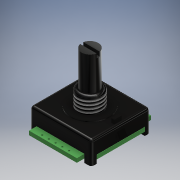
# Autodesk Inventor part: Bourns ACE 128
Saved by Autodesk Inventor 2017 SP1 (Build 210196100, 196)
## iProperties
Created: 2018-01-09
Part Number: Bourns ACE 128
Material: ABS Plastic
Document SubType Name: Modeling
Designer: Zach
Density: 1.06 g/cm^3
Appearance: Glossy - Black
Author: Zach
Autodesk Inventor part; units mm, degrees
ref_plane "YZ Plane" through (0, 0, 0) normal (1, 0, 0) x (0, 1, 0)
ref_plane "XZ Plane" through (0, 0, 0) normal (0, 1, 0) x (-1, 0, 0)
ref_plane "XY Plane" through (0, 0, 0) normal (0, 0, 1) x (1, 0, 0)
sketch "Sketch1" plane through (0, 0, 0) normal (0, 0, 1) x (1, 0, 0)
  line L0 (0, 0) -> (18.04, 0)
  line L1 (18.04, 0) -> (18.04, 27.94) construction
  line L2 (18.04, 27.94) -> (0, 27.94)
  line L3 (0, 27.94) -> (0, 0) construction
  circle A0 centre (9.02, 26.94) radius 0.32
  circle A1 centre (6.48, 26.94) radius 0.32
  circle A2 centre (3.94, 26.94) radius 0.32
  circle A3 centre (11.56, 26.94) radius 0.32
  circle A4 centre (14.1, 26.94) radius 0.32
  circle A5 centre (9.02, 1) radius 0.32
  circle A6 centre (6.48, 1) radius 0.32
  circle A7 centre (3.94, 1) radius 0.32
  circle A8 centre (11.56, 1) radius 0.32
  circle A9 centre (14.1, 1) radius 0.32
  line L4 (-2.665, 23.07) -> (20.705, 23.07) construction
  line L5 (20.705, 23.07) -> (20.705, 4.87) construction
  line L6 (20.705, 4.87) -> (-2.665, 4.87) construction
  line L7 (-2.665, 4.87) -> (-2.665, 23.07) construction
  line L8 (0, 27.94) -> (0, 23.07)
  line L9 (0, 23.07) -> (-2.665, 23.07)
  line L10 (-2.665, 23.07) -> (-2.665, 4.87)
  line L11 (-2.665, 4.87) -> (0, 4.87)
  line L12 (0, 0) -> (0, 4.87)
  line L13 (18.04, 0) -> (18.04, 4.87)
  line L14 (18.04, 4.87) -> (20.705, 4.87)
  line L15 (20.705, 4.87) -> (20.705, 23.07)
  line L16 (20.705, 23.07) -> (18.04, 23.07)
  line L17 (18.04, 23.07) -> (18.04, 27.94)
  point P0 (9.02, 27.94)
  point P1 (9.02, 23.07)
  point P2 (18.04, 13.97)
  point P3 (20.705, 13.97)
  dimension "d0" = 18.04
  dimension "d1" = 27.94
  dimension "d2" = 0.64
  dimension "d3" = 0.64
  dimension "d4" = 2.54
  dimension "d5" = 0.64
  dimension "d6" = 0.64
  dimension "d7" = 0.64
  dimension "d8" = 2.54
  dimension "d9" = 2.54
  dimension "d10" = 2.54
  dimension "d11" = 1
  dimension "d12" = 0.64
  dimension "d13" = 0.64
  dimension "d14" = 2.54
  dimension "d15" = 0.64
  dimension "d16" = 0.64
  dimension "d17" = 0.64
  dimension "d18" = 2.54
  dimension "d19" = 2.54
  dimension "d20" = 2.54
  dimension "d21" = 1
  dimension "d24" = 23.37
  dimension "d25" = 18.2
  constraints: 36 end point, 10 centre point, 9 horizontal alignment, 8 point on line, 4 collinear, 4 midpoint, 4 parallel, 4 perpendicular, 3 vertical alignment, 2 horizontal
  measures "d0" distance of L2.end L1.end
  measures "d1" distance of L1.end L0.end
  measures "d2" diameter of A0
  measures "d3" diameter of A1
  measures "d4" distance of A0.centre A1.centre
  measures "d5" diameter of A2
  measures "d6" diameter of A3
  measures "d7" diameter of A4
  measures "d8" distance of A3.centre A0.centre
  measures "d9" distance of A4.centre A3.centre
  measures "d10" distance of A2.centre A1.centre
  measures "d11" distance from line of L2 A2.centre
  measures "d12" diameter of A5
  measures "d13" diameter of A6
  measures "d14" distance of A5.centre A6.centre
  measures "d15" diameter of A7
  measures "d16" diameter of A8
  measures "d17" diameter of A9
  measures "d18" distance of A8.centre A5.centre
  measures "d19" distance of A9.centre A8.centre
  measures "d20" distance of A7.centre A6.centre
  measures "d21" distance from line of L0 A5.centre
  measures "d24" distance of L5.end L6.end
  measures "d25" distance of L4.end L5.end
extrude "Extrusion1" add sketch "Sketch1" along normal blind 1.5
sketch "Sketch2" plane through (0, 0, 1.5) normal (0, 0, 1) x (1, 0, 0)
  line L0 (-2.565, 25.07) -> (20.605, 25.07)
  line L1 (20.605, 25.07) -> (20.605, 2.87)
  line L2 (20.605, 2.87) -> (-2.565, 2.87)
  line L3 (-2.565, 2.87) -> (-2.565, 25.07)
  line L4 (-2.665, 23.07) -> (-2.665, 4.87) projected
  line L5 (20.705, 4.87) -> (20.705, 23.07) projected
  line L6 (18.04, 27.94) -> (0, 27.94) projected
  point P0 (0, 0)
  point P1 (9.02, 25.07)
  point P2 (9.02, 27.94)
  dimension "d27" = 22.2
  dimension "d30" = 0.1
  constraints: 8 end point, 2 midpoint, 2 parallel, 1 horizontal, 1 perpendicular, 1 vertical alignment
  measures "d27" distance of L0.end L1.end
  measures "d30" distance between parallel lines of L5 L1
extrude "Extrusion2" add sketch "Sketch2" along normal blind 5.51
sketch "Sketch3" plane through (0, 0, 1.5) normal (0, 0, -1) x (-1, 0, 0)
  line L0 (0, 23.07) -> (2.565, 23.07) projected
  line L1 (2.565, 23.07) -> (2.565, 25.07) projected
  line L2 (2.565, 25.07) -> (0, 25.07) projected
  line L3 (0, 25.07) -> (0, 23.07) projected
  line L4 (0, 4.87) -> (0, 2.87) projected
  line L5 (0, 2.87) -> (2.565, 2.87) projected
  line L6 (2.565, 2.87) -> (2.565, 4.87) projected
  line L7 (2.565, 4.87) -> (0, 4.87) projected
  line L8 (-20.605, 23.07) -> (-18.04, 23.07) projected
  line L9 (-18.04, 23.07) -> (-18.04, 25.07) projected
  line L10 (-18.04, 25.07) -> (-20.605, 25.07) projected
  line L11 (-20.605, 25.07) -> (-20.605, 23.07) projected
  line L12 (-18.04, 2.87) -> (-18.04, 4.87) projected
  line L13 (-18.04, 4.87) -> (-20.605, 4.87) projected
  line L14 (-20.605, 4.87) -> (-20.605, 2.87) projected
  line L15 (-20.605, 2.87) -> (-18.04, 2.87) projected
  point P0 (0, 0)
extrude "Extrusion3" add sketch "Sketch3" along normal blind 3
sketch "Sketch4" plane through (0, 0, 7.01) normal (0, 0, 1) x (1, 0, 0)
  circle A0 centre (9.02, 13.97) radius 4.5
  line L0 (20.605, 25.07) -> (-2.565, 25.07) construction
  line L1 (-2.565, 25.07) -> (-2.565, 2.87) construction
  line L2 (-2.565, 2.87) -> (20.605, 2.87) construction
  line L3 (20.605, 2.87) -> (20.605, 25.07) construction
  point P0 (0, 0)
  point P1 (9.02, 25.07)
  point P2 (20.605, 13.97)
  dimension "d33" = 9
  constraints: 2 midpoint, 1 centre point, 1 horizontal alignment, 1 vertical alignment
  measures "d33" diameter of A0
extrude "Extrusion4" add sketch "Sketch4" along normal blind 6.35
sketch "Sketch5" plane through (9.02, 13.97, 13.36) normal (0, 0, 1) x (1, 0, 0)
  circle A0 centre (0, 0) radius 3.16
  circle A1 centre (0, 0) radius 4.5 construction
  point P0 (-9.02, -13.97)
  dimension "d36" = 6.32
  constraints: 1 centre point, 1 coincident
  measures "d36" diameter of A0
extrude "Extrusion5" add sketch "Sketch5" along normal blind 12.7
sketch "Sketch6" plane through (9.02, 13.97, 26.06) normal (0, 0, 1) x (1, 0, 0)
  line L0 (-3.16, 0.595) -> (3.16, 0.595)
  line L1 (3.16, 0.595) -> (3.16, -0.595)
  line L2 (3.16, -0.595) -> (-3.16, -0.595)
  line L3 (-3.16, -0.595) -> (-3.16, 0.595)
  circle A0 centre (0, 0) radius 3.16 construction
  point P0 (-9.02, -13.97)
  point P1 (3.16, 0)
  point P2 (0, 0.595)
  dimension "d39" = 1.19
  constraints: 8 end point, 2 horizontal alignment, 2 midpoint, 2 parallel, 1 horizontal, 1 perpendicular, 1 vertical alignment, 1 other
  measures "d39" distance of L0.end L1.end
extrude "Extrusion6" cut sketch "Sketch6" against normal blind 1.6
thread "Thread1" size "M9x1.25" class "6g" standard "ANSI Metric M Profile" full length
fillet "Fillet1" radius 1 1 edges at (4.52, 13.97, 13.36)
fillet "Fillet2" radius 1 4 edges at (20.605, 2.87, 2.755) (-2.565, 2.87, 2.755) (-2.565, 25.07, 2.755) (20.605, 25.07, 2.755)
fillet "Fillet3" radius 1 8 edges at (-2.2721, 24.7771, 7.01) (-2.565, 13.97, 7.01) (-2.2721, 3.1629, 7.01) (9.02, 2.87, 7.01) (20.3121, 3.1629, 7.01) (20.605, 13.97, 7.01) (20.3121, 24.7771, 7.01) (9.02, 25.07, 7.01)
ref_plane "Work Plane1" through (0, 13.97, 1.5) normal (0, 1, 0) x (1, 0, 0)
sketch "Sketch8" plane through (0, 13.97, 1.5) normal (0, 1, 0) x (1, 0, 0)
  line L0 (19.605, -1.51) -> (21.605, -1.51)
  line L1 (19.605, 3) -> (19.605, -4.51) construction
  line L2 (19.605, -1.51) -> (19.605, -5.51)
  line L3 (0, 1.5) -> (18.04, 1.5) construction
  line L4 (9.02, 1.5) -> (9.02, -5.51) construction
  line L5 (19.605, -5.51) -> (-1.565, -5.51) construction
  line L6 (21.605, -1.51) -> (19.605, -5.51)
  line L7 (-1.565, -1.51) -> (-3.565, -1.51)
  line L8 (-1.565, -1.51) -> (-1.565, -5.51)
  line L9 (-3.565, -1.51) -> (-1.565, -5.51)
  dimension "d47" = 2
  dimension "d48" = 4
  constraints: 14 end point, 3 symmetric about line, 2 vertical, 1 horizontal, 1 midpoint, 1 point on line
  measures "d47" distance of L0.start L0.end
  measures "d48" distance of L2.end L0.start
extrude "Extrusion7" add sketch "Sketch8" along normal mid plane 2.79
sketch "Sketch9" plane through (0, 13.97, 1.5) normal (0, 1, 0) x (1, 0, 0)
  line L0 (-1.565, -5.51) -> (19.605, -5.51) projected
  line L1 (19.605, -5.51) -> (18.415, -5.51)
  line L2 (18.415, -5.51) -> (18.415, -7.03)
  line L3 (18.415, -7.03) -> (19.605, -7.03)
  line L4 (19.605, -7.03) -> (19.605, -5.51)
  point P0 (0, 1.5)
  dimension "d51" = 1.52
  dimension "d52" = 1.19
  constraints: 8 end point, 2 parallel, 1 horizontal, 1 perpendicular
  measures "d51" distance of L2.end L1.end
  measures "d52" distance of L2.end L3.end
extrude "Extrusion8" add sketch "Sketch9" along normal mid plane 2.79
sketch "Sketch10" plane through (0, 0, 7.01) normal (0, 0, 1) x (1, 0, 0)
  circle A0 centre (9.02, 13.97) radius 4.5 projected
  circle A1 centre (9.02, 13.97) radius 7.35
  point P0 (0, 0)
  dimension "d55" = 14.7
  constraints: 1 centre point, 1 coincident
  measures "d55" diameter of A1
extrude "Extrusion9" add sketch "Sketch10" along normal blind 0.25 contours A0 | A1
equation "\"d2\" = d5"
equation "\"d3\" = d5"
equation "\"d6\" = d5"
equation "\"d7\" = d5"
equation "\"d12\" = d5"
equation "\"d13\" = d5"
equation "\"d15\" = d5"
equation "\"d16\" = d5"
equation "\"d17\" = d5"
equation "\"d21\" = d11"
body "Solid1"
